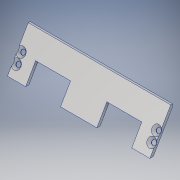
# Autodesk Inventor part: Przod
Saved by Autodesk Inventor 2019 (Build 230136000, 136)
## iProperties
Created: 2022-01-30
Part Number: Przod
Material: Aluminium 6061
Document SubType Name: Modeling
Designer: Michał
Density: 2.7 g/cm^3
Appearance: Aluminium — płaski
Mass: 10.9411 g
Surface Area: 48.0142 cm^2
Volume: 4.05227 cm^3
Author: Michał
Autodesk Inventor part; units mm, degrees
ref_plane "YZ Plane" through (0, 0, 0) normal (1, 0, 0) x (0, 1, 0)
ref_plane "XZ Plane" through (0, 0, 0) normal (0, 1, 0) x (-1, 0, 0)
ref_plane "XY Plane" through (0, 0, 0) normal (0, 0, 1) x (1, 0, 0)
sketch "Szkic1" plane through (0, 0, 0) normal (1, 0, 0) x (0, 1, 0)
  line L0 (0, 0) -> (0, -2.3094)
  line L1 (0, -2.3094) -> (23, -15.5885)
  line L2 (24.75, -14.2894) -> (0, 0)
  line L3 (23, -15.5885) -> (24.75, -15.5885)
  line L4 (24.75, -15.5885) -> (24.75, -14.2894)
  dimension "d0" = 60
  dimension "d1" = 2
  dimension "d2" = 1.75
  dimension "d3" = 23
  constraints: 10 end point, 1 horizontal, 1 parallel, 1 perpendicular, 1 vertical
  measures "d0" angle of L1 L0
  measures "d1" distance between parallel lines of L2 L1
  measures "d2" distance of L1.end L3.end
  measures "d3" distance from line of L0 L1.end
extrude "Wyciągnięcie proste1" add sketch "Szkic1" along normal blind 98
sketch "Szkic2" plane through (98, 24.75, -15.5885) normal (0, 0, -1) x (-1, 0, 0)
  line L0 (98, -24.75) -> (0, -24.75) construction
  line L1 (12.5, -24.75) -> (36.5, -24.75)
  line L2 (36.5, -24.75) -> (36.5, -12.75)
  line L3 (36.5, -12.75) -> (12.5, -12.75)
  line L4 (12.5, -12.75) -> (12.5, -24.75)
  line L5 (49, -24.75) -> (49, 0) construction
  line L6 (98, 0) -> (0, 0) construction
  line L7 (85.5, -24.75) -> (61.5, -24.75)
  line L8 (61.5, -24.75) -> (61.5, -12.75)
  line L9 (61.5, -12.75) -> (85.5, -12.75)
  line L10 (85.5, -12.75) -> (85.5, -24.75)
  line L11 (0, -24.75) -> (0, -1.75) construction
  dimension "d6" = 12
  dimension "d7" = 24
  dimension "d8" = 12.5
  constraints: 18 end point, 4 symmetric about line, 2 midpoint, 2 parallel, 1 horizontal, 1 perpendicular, 1 point on line
  measures "d6" distance of L3.end L1.start
  measures "d7" distance of L2.end L3.end
  measures "d8" distance between parallel lines of L11 L4
extrude "Wyciągnięcie proste2" cut sketch "Szkic2" against normal through all
sketch "Szkic3" plane through (0, 24.75, -14.2894) normal (0, 0.5, 0.8660254) x (1, 0, 0)
  line L0 (0, -28.5788) -> (12.5, -28.5788) construction
  line L1 (2.4, -28.5788) -> (2.4, -14.6241) construction
  line L2 (0, 0) -> (0, -28.5788) construction
  line L3 (0, -27.4241) -> (12.5, -27.4241) construction
  line L4 (36.5, -28.5788) -> (61.5, -28.5788) construction
  line L5 (49, -28.5788) -> (49, 0.6495) construction
  line L6 (0, 0.6495) -> (98, 0.6495) construction
  point P0 (2.4, -21.1241)
  point P1 (95.6, -14.6241)
  point P2 (95.6, -21.1241)
  dimension "d11" = 2.4
  dimension "d12" = 6.3
  dimension "d13" = 12.8
  constraints: 4 end point, 2 midpoint, 2 point on line, 2 symmetric about line, 1 coincident, 1 vertical
  measures "d11" distance between parallel lines of L2 L1
  measures "d12" distance from line of point (2.4, -21.124) L3
  measures "d13" distance from line of L1.end L3
hole "Otwór1" at (2.4, 12.0851, -6.9774) at (2.4, 6.456, -3.7274) at (95.6, 12.0851, -6.9774) at (95.6, 6.456, -3.7274) direction (0, -0.5, -0.8660254) diameter 3.2 depth 5 tip angle 118 countersink diameter 6.3 countersink angle 84.225 clearance for "Śruba ze łbem stożkowym ISO 2009/7046" size "M3" standard "ISO"
